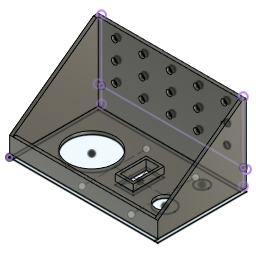
12v-socket-mounting-bracket_v7 (Autodesk Fusion 360 design; units mm, degrees)
Autodesk Fusion 360 part; units mm, degrees
sketch "Skizze1" plane through (0, 0, 0) normal (0, 0, 1) x (1, 0, 0) in component "Montagewinkel"
  line L0 (0, 0) -> (92, 0)
  line L1 (92, 0) -> (92, 55)
  line L2 (92, 55) -> (0, 55)
  line L3 (0, 55) -> (0, 0)
  line L4 (2, 2) -> (90, 2)
  line L5 (90, 2) -> (90, 53)
  line L6 (90, 53) -> (2, 53)
  line L7 (2, 53) -> (2, 2)
  line L8 (2, 53) -> (2, 55)
  line L9 (90, 53) -> (90, 55)
  line L10 (2, 2) -> (2, 0)
  line L11 (90, 2) -> (90, 0)
  circle A0 centre (23.5, 27.5) radius 14.5
  circle A1 centre (74.5, 22) radius 6
  circle A2 centre (74.5, 45) radius 4
  line L12 (38, 47) -> (38, 7) construction
  line L13 (68.5, 47) -> (68.5, 7) construction
  line L14 (68.5, 27.5) -> (38, 27.5) construction
  line L15 (57.25, 19.5) -> (49.25, 19.5)
  line L16 (49.25, 19.5) -> (49.25, 35.5)
  line L17 (49.25, 35.5) -> (57.25, 35.5)
  line L18 (57.25, 35.5) -> (57.25, 19.5)
  line L19 (57.25, 19.5) -> (49.25, 35.5) construction
  line L20 (49.25, 19.5) -> (57.25, 35.5) construction
  line L21 (58.85, 17.9) -> (47.65, 17.9)
  line L22 (47.65, 17.9) -> (47.65, 37.1)
  line L23 (47.65, 37.1) -> (58.85, 37.1)
  line L24 (58.85, 37.1) -> (58.85, 17.9)
  point P0 (53.25, 27.5)
  dimension "d1" = 92
  dimension "d2" = 55
  dimension "d3" = -2
  dimension "d4" = 29
  dimension "d5" = 23.5
  dimension "d6" = 27.5
  dimension "d7" = 12
  dimension "d8" = 22
  dimension "d9" = 17.5
  dimension "d10" = 8
  dimension "d11" = 10
  dimension "d12" = 17.5
  dimension "d13" = 27.5
  dimension "d14" = 8
  dimension "d15" = 16
  dimension "d16" = -1.6
  constraint horizontal L0
  constraint vertical L1
  constraint horizontal L2
  constraint vertical L3
  constraint coincident L0.start L3.end
  constraint coincident L2 L8.end
  constraint perpendicular L2 L8
  constraint coincident L2 L9.end
  constraint perpendicular L2 L9
  constraint coincident L0 L10.end
  constraint perpendicular L0 L10
  constraint coincident L0 L11.end
  constraint perpendicular L0 L11
  constraint vertical L12
  constraint tangent A0 L12
  constraint vertical L13
  constraint tangent A1 L13
  constraint coincident L13 L14.start
  constraint coincident L12 L14.end
  constraint perpendicular L12 L14
  constraint horizontal L15
  constraint perpendicular L15 L16
  constraint parallel L15 L17
  constraint parallel L16 L18
  constraint coincident L19 P0
  constraint coincident L20 P0
  constraint midpoint L14 P0
  measures "d1" distance of L0.start L0.end
  measures "d2" distance of L0.start L2.end
  measures "d4" diameter of A0
  measures "d5" distance of L3 A0.centre
  measures "d6" distance of L2 A0.centre
  measures "d7" diameter of A1
  measures "d8" distance of L0 A1.centre
  measures "d9" distance of L1 A1.centre
  measures "d10" diameter of A2
  measures "d11" distance of L2 A2.centre
  measures "d12" distance of L1 A2.centre
  measures "d13" distance of L2 L14
  measures "d14" distance of L16.end L17.end
  measures "d15" distance of L15.end L16.end
extrude "Extrusion1" add sketch "Skizze1" along normal blind 2 contours L4 L5 L6 L7 in component "Montagewinkel"
extrude "Extrusion3" add sketch "Skizze1" along normal blind 6 contours L21 L22 L23 L24 in component "Montagewinkel"
extrude "Extrusion4" add sketch "Skizze1" along normal blind 50 contours L0 L2 L3 L7 L8 L10 | L0 L1 L2 L5 L9 L11 | L2 L6 L8 L9 in component "Montagewinkel"
extrude "Extrusion5" add sketch "Skizze1" along normal blind 12 contours L0 L4 L10 L11 in component "Montagewinkel"
chamfer "Fase1" distance 52 distance2 38 2 edges at (1, 0, 50) (91, 0, 50) measured on face at (31.3333, 54.3333, 50) measured on face at (31.3333, 54.3333, 50) in component "Montagewinkel"
chamfer "Fase2" distance 2 angle 45 3 edges at (46, 0, 0) (0, 27.5, 0) (92, 27.5, 0) in component "Montagewinkel"
sketch "Skizze2" plane through (0, 55, 0) normal (0, 1, 0) x (-1, 0, 0) in component "Montagewinkel"
  line L0 (-92, 2) -> (-90, 0)
  line L1 (-90, 0) -> (-2, 0)
  line L2 (-2, 0) -> (0, 2)
  line L3 (0, 2) -> (0, 50)
  line L4 (0, 50) -> (-92, 50)
  line L5 (-92, 50) -> (-92, 2)
  line L6 (0, 12) -> (-2, 12)
  line L7 (-2, 12) -> (-90, 12)
  line L8 (-90, 12) -> (-92, 12)
  line L9 (-2, 2) -> (-2, 50)
  line L10 (-90, 2) -> (-90, 50)
  circle A0 centre (-80, 19) radius 1.8
  circle A1 centre (-63, 19) radius 1.8
  circle A2 centre (-80, 31) radius 1.8
  circle A3 centre (-63, 31) radius 1.8
  circle A4 centre (-46, 19) radius 1.8
  circle A5 centre (-29, 19) radius 1.8
  circle A6 centre (-12, 19) radius 1.8
  circle A7 centre (-46, 31) radius 1.8
  circle A8 centre (-29, 31) radius 1.8
  circle A9 centre (-12, 31) radius 1.8
  circle A10 centre (-80, 43) radius 1.8
  circle A11 centre (-63, 43) radius 1.8
  circle A12 centre (-46, 43) radius 1.8
  circle A13 centre (-29, 43) radius 1.8
  circle A14 centre (-12, 43) radius 1.8
  dimension "d30" = 3.6
  dimension "d31" = 10
  dimension "d32" = 7
  dimension "d36" = 68
  dimension "d37" = 24
  measures "d30" diameter of A0
  measures "d31" distance of L10 A0.centre
  measures "d32" distance of L7 A0.centre
extrude "Extrusion6" cut sketch "Skizze2" against normal blind 2 contours A0 | A1 | A2 | A3 | A4 | A5 | A6 | A7 | A8 | A9 | A10 | A11 | A12 | A13 | A14 in component "Montagewinkel"
component "Montagewinkel" placed x (1, 0, 0) y (0, 1, 0) z (0, 0, 1) at (0, 0, 0)
equation "d5 = ( 37 / 2 ) * 1 mm + 5 mm"
equation "d6 = ( 55 / 2 ) * 1 mm"
equation "d8 = 5 mm + ( 34 / 2 ) * 1 mm"
equation "d9 = 5 mm + ( 25 / 2 ) * 1 mm"
equation "d11 = 5 mm + 5 mm"
equation "d13 = ( 55 / 2 ) * 1 mm"
named bodies: "Montagewinkel"
